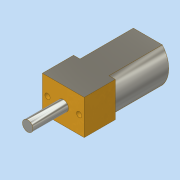
# Autodesk Inventor part: MicroGearMotor
Saved by Autodesk Inventor 2017.3 (Build 213256000, 256)
## iProperties
Created: 2018-07-04
Part Number: MicroGearMotor
Material: Brass, Soft Yellow, Welded
Document SubType Name: Modeling
Designer: Derek Wider
Density: 8.5 g/cm^3
Appearance: Weld - Brass
Author: Derek Wider
Autodesk Inventor part; units mm, degrees
ref_plane "YZ Plane" through (0, 0, 0) normal (1, 0, 0) x (0, 1, 0)
ref_plane "XZ Plane" through (0, 0, 0) normal (0, 1, 0) x (-1, 0, 0)
ref_plane "XY Plane" through (0, 0, 0) normal (0, 0, 1) x (1, 0, 0)
sketch "Sketch1" plane through (0, 0, 0) normal (0, 0, 1) x (1, 0, 0)
  line L0 (0, 0) -> (11.9253, 0)
  line L1 (11.9253, 0) -> (11.9253, 9.9314)
  line L2 (11.9253, 9.9314) -> (0, 9.9314)
  line L3 (0, 9.9314) -> (0, 0)
  dimension "d0" = 11.9253
  dimension "d1" = 9.9314
  constraints: 8 end point, 2 parallel, 1 horizontal, 1 perpendicular
  measures "d0" distance of L1.end L2.end
  measures "d1" distance of L0.end L1.end
extrude "Extrusion1" add sketch "Sketch1" along normal blind 8.89
sketch "Sketch2" plane through (0, 0, 8.89) normal (0, 0, 1) x (1, 0, 0)
  circle A0 centre (5.9626, 4.9657) radius 1.5
  line L0 (11.9253, 9.9314) -> (0, 9.9314) construction
  line L1 (0, 9.9314) -> (0, 0) construction
  point P0 (5.9626, 9.9314)
  point P1 (0, 4.9657)
  dimension "d4" = 3
  constraints: 2 midpoint, 1 centre point, 1 horizontal alignment, 1 vertical alignment
  measures "d4" diameter of A0
extrude "Extrusion2" add sketch "Sketch2" along normal blind 10.16
sketch "Sketch3" plane through (0, 0, 8.89) normal (0, 0, 1) x (1, 0, 0)
  circle A0 centre (10.4711, 4.9657) radius 0.762
  circle A1 centre (1.4541, 4.9657) radius 0.762
  line L0 (1.4541, 4.9657) -> (0, 4.9657) construction
  line L1 (0, 9.9314) -> (0, 0) construction
  line L2 (10.4711, 4.9657) -> (11.9253, 4.9657) construction
  line L3 (11.9253, 0) -> (11.9253, 9.9314) construction
  dimension "d7" = 9.017
  dimension "d8" = 1.524
  constraints: 4 end point, 3 midpoint, 2 centre point, 1 coincident, 1 collinear, 1 equal radius, 1 horizontal, 1 horizontal alignment, 1 point on line
  measures "d7" distance of L2.start L0.start
  measures "d8" diameter of A1
extrude "Extrusion3" cut sketch "Sketch3" against normal blind 7.62
sketch "Sketch4" plane through (0, 0, 0) normal (0, 0, -1) x (-1, 0, 0)
  line L0 (0, 0) -> (-11.9253, 0) construction
  line L1 (0, 9.9314) -> (0, 0) construction
  line L2 (-11.9253, 9.9314) -> (0, 9.9314) construction
  line L3 (-11.9253, 0) -> (-11.9253, 9.9314) construction
  line L4 (-11.9253, 9.9314) -> (0, 9.9314) projected
  line L5 (-1.8351, 9.9314) -> (-10.0901, 9.9314)
  line L6 (0, 0) -> (-11.9253, 0) projected
  line L7 (-1.8351, 0) -> (-10.0901, 0)
  arc A0 (-10.0901, 9.9314) -> (-10.0901, 0) centre (-4.2894, 4.9657) ccw
  arc A1 (-1.8351, 0) -> (-1.8351, 9.9314) centre (-7.6359, 4.9657) ccw
  line L8 (0, 9.9314) -> (0, 0) projected
  line L9 (-11.9253, 0) -> (-11.9253, 9.9314) projected
  dimension "d11" = 8.255
  constraints: 4 end point, 4 point on circle, 4 point on line, 2 centre point, 2 tangent, 2 vertical alignment, 1 equal radius, 1 parallel
  measures "d11" distance of L5.start L5.end
extrude "Extrusion4" add sketch "Sketch4" along normal blind 15.24 contours L4 A1 L6 A0
sketch "Sketch5" plane through (0, 0, -15.24) normal (0, 0, -1) x (-1, 0, 0)
  circle A0 centre (-5.9626, 4.9657) radius 1.5 construction
  circle A1 centre (-5.9626, 4.9657) radius 1.5 projected
  circle A2 centre (-5.9626, 4.9657) radius 2.2225
  point P0 (0, 0)
  dimension "d14" = 4.445
  constraints: 1 centre point, 1 coincident
  measures "d14" diameter of A2
extrude "Extrusion5" add sketch "Sketch5" along normal blind 1.27 contours A1 | A2
body "Solid1"
